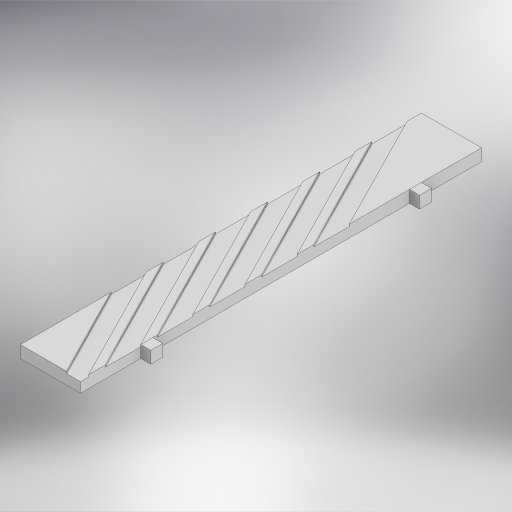
# Autodesk Inventor part: Module Cradle V1
Saved by Autodesk Inventor 2024 (Build 280153000, 153)
## iProperties
Created: 2024-03-20
Part Number: Module Cradle V1
Material: Generic
Document SubType Name: Modeling
Designer: cfang
Density: 1 g/cm^3
Appearance: Default
Author: cfang
Autodesk Inventor part; units mm, degrees
ref_plane "YZ Plane" through (0, 0, 0) normal (1, 0, 0) x (0, 1, 0)
ref_plane "XZ Plane" through (0, 0, 0) normal (0, 1, 0) x (-1, 0, 0)
ref_plane "XY Plane" through (0, 0, 0) normal (0, 0, 1) x (1, 0, 0)
sketch "Sketch3" plane through (0, 0, 0) normal (0, 1, 0) x (-1, 0, 0)
  line L0 (-15, -100) -> (15, -100)
  line L1 (15, -100) -> (15, 100)
  line L2 (15, 100) -> (-15, 100)
  line L3 (-15, 100) -> (-15, -100)
  line L4 (-15, -100) -> (15, 100) construction
  line L5 (15, -100) -> (-15, 100) construction
  point P0 (0, 0)
  dimension "d7" = 30
  dimension "d8" = 200
  constraints: 12 end point, 2 midpoint, 2 parallel, 1 horizontal, 1 perpendicular
  measures "d7" distance of L1.end L2.end
  measures "d8" distance of L0.end L1.end
extrude "Extrusion2" add sketch "Sketch3" along normal blind 6
sketch "Sketch4" plane through (0, 6, 0) normal (0, 1, 0) x (1, 0, 0)
  line L0 (-15, 100) -> (-15, -100) projected
  line L1 (-15, -54.7432) -> (15, -113.6215)
  line L2 (15, -100) -> (15, 100) projected
  line L3 (-15, -37.1217) -> (15, -96)
  line L4 (-15, -100) -> (15, -100) projected
  line L5 (-15, -28.7432) -> (15, -87.6215)
  line L6 (-15, -11.1217) -> (15, -70)
  line L7 (-15, -2.7432) -> (15, -61.6215)
  line L8 (-15, 14.8783) -> (15, -44)
  line L9 (-15, 23.2568) -> (15, -35.6215)
  line L10 (-15, 40.8783) -> (15, -18)
  line L11 (-15, 49.2568) -> (15, -9.6215)
  line L12 (-15, 66.8783) -> (15, 8)
  line L13 (-15, 75.2568) -> (15, 16.3785)
  line L14 (-15, 92.8783) -> (15, 34)
  point P0 (0, 0)
  point P1 (15, -50.386)
  point P2 (8.0595, -100)
  point P3 (15, 34)
  point P4 (15, 8)
  point P5 (15, -18)
  point P6 (15, -44)
  point P7 (15, -70)
  dimension "d11" = 27
  dimension "d12" = 8
  dimension "d23" = 4
  dimension "d26" = 26
  constraints: 24 end point, 4 point on line, 1 parallel, 1 vertical, 30 other
  measures "d11" angle of L0 L1
  measures "d12" distance between parallel lines of L1 L3
  measures "d23" distance from line of L4 L3.end
  measures "d26" distance of L1.start L5.start
extrude "Extrusion3" cut sketch "Sketch4" against normal blind 1 contours L14 L2 L13 L0 | L12 L2 L11 L0 | L10 L2 L9 L0 | L8 L2 L7 L0 | L6 L2 L5 L0 | L3 L2 L4 L1 L0
sketch "Sketch6" plane through (15, 0, 100) normal (1, 0, 0) x (0, 0, -1)
  line L0 (200, 0) -> (0, 0) projected
  line L1 (30, 0) -> (36, 0)
  line L2 (36, 0) -> (36, 5.9996)
  line L3 (36, 5.9996) -> (30, 5.9996)
  line L4 (30, 5.9996) -> (30, 0)
  line L5 (164, 0) -> (170, 0)
  line L6 (170, 0) -> (170, 5.9996)
  line L7 (170, 5.9996) -> (164, 5.9996)
  line L8 (164, 5.9996) -> (164, 0)
  line L9 (0, 0) -> (200, 0) projected
  point P0 (100, 0)
  point P1 (36, 2.9998)
  point P2 (100, 0)
  point P3 (100, 0)
  point P4 (170, 0)
  dimension "d34" = 6
  dimension "d35" = 64
  dimension "d36" = 6
  dimension "d37" = 64
  constraints: 16 end point, 4 parallel, 2 horizontal, 2 midpoint, 2 perpendicular, 2 point on line, 2 other
  measures "d34" distance of L2.end L3.end
  measures "d35" horizontal distance of point (36, 3) point (100, 0)
  measures "d36" distance of L6.end L7.end
  measures "d37" distance from line of point (100, 0) L8
extrude "Extrusion4" add sketch "Sketch6" along normal blind 5
equation "\"d36\" = d34"
equation "\"d37\" = d35"
body "Solid2"
